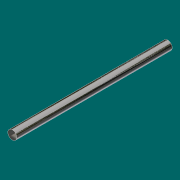
# Autodesk Inventor part: 2.25 bar x 3.25ft
Saved by Autodesk Inventor 2017 (Build 210142000, 142)
## iProperties
Created: 2018-01-23
Part Number: 2.25 bar x 3.25ft
Material: Steel, Alloy
Document SubType Name: Modeling
Designer: Graeme_Van_Dongen
Density: 7.73 g/cm^3
Appearance: Semi-Polished
Mass: 19642.7 g
Surface Area: 1829.85 cm^2
Volume: 2541.09 cm^3
Author: Graeme_Van_Dongen
Autodesk Inventor part; units mm, degrees
ref_plane "YZ Plane" through (0, 0, 0) normal (1, 0, 0) x (0, 1, 0)
ref_plane "XZ Plane" through (0, 0, 0) normal (0, 1, 0) x (-1, 0, 0)
ref_plane "XY Plane" through (0, 0, 0) normal (0, 0, 1) x (1, 0, 0)
sketch "Sketch1" plane through (0, 0, 0) normal (0, 0, 1) x (1, 0, 0)
  circle A0 centre (0, 0) radius 28.575
  dimension "d0" = 57.15
  constraints: 1 centre point, 1 coincident
  measures "d0" diameter of A0
extrude "Extrusion1" add sketch "Sketch1" along normal blind 990.6
body "Solid1"
